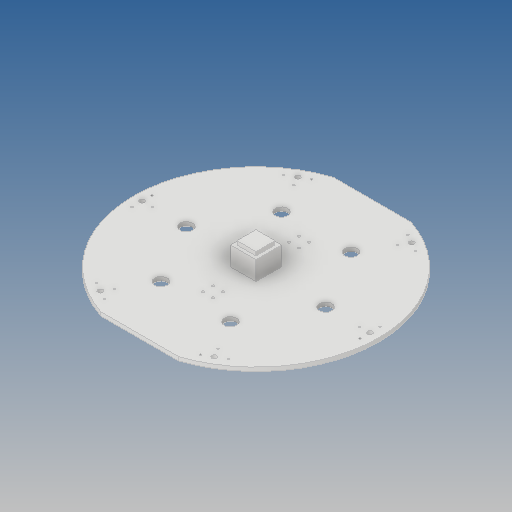
# Autodesk Inventor part: 1
Saved by Autodesk Inventor 2020 (Build 240168000, 168)
## iProperties
Created: 2019-09-06
Part Number: 1
Material: Пластик АБС
Document SubType Name: Modeling
Designer: Iliga
Density: 1.06 g/cm^3
Appearance: Гладкий — белый
Mass: 236.83 g
Surface Area: 2382.33 cm^2
Volume: 236.83 cm^3
Author: Iliga
Autodesk Inventor part; units mm, degrees
ref_plane "РабПлоскость1" through (0, -35, 0) normal (0, 1, 0) x (-1, 0, 0)
ref_plane "РабПлоскость7" through (100, -35, 0) normal (0, -1, 0) x (1, 0, 0)
sketch "Эскиз121" plane through (0, 0, 0) normal (0, 0, 1) x (1, 0, 0)
  line L0 (-100, 0) -> (0, 0)
  line L1 (0, 147.6791) -> (0, -62.3209)
  line L2 (0, 3) -> (-96.9536, 3)
  line L3 (-78.4857, 57) -> (0, 57)
  line L4 (0, 0) -> (0, 3)
  line L5 (0, 57) -> (0, 63)
  line L6 (0, 60) -> (-80, 60)
  arc A0 (-80, 60) -> (-100, 0) centre (0, 0) ccw
  arc A1 (-78.4857, 57) -> (-96.9536, 3) centre (0, 0) ccw
  dimension "d674" = 3
  dimension "d680" = 3
  dimension "d681" = 60
  dimension "d683" = 100
  dimension "d684" = 97
  constraints: 14 end point, 4 point on circle, 3 horizontal, 2 centre point, 2 coincident, 2 perpendicular, 2 point on line, 1 collinear, 1 midpoint, 1 parallel, 1 vertical
  measures "d674" distance between parallel lines of L0 L2
  measures "d680" distance between parallel lines of L3 L6
  measures "d681" distance between parallel lines of L0 L6
  measures "d683" radius of A0
  measures "d684" radius of A1
revolve "Вращение3" add sketch "Эскиз121" angle 180 mid plane about axis through (0, 147.6791, 0) along (0, -1, 0) contours A0 L6 L1 L3 A1 L2 L0
sketch "Эскиз124" plane through (0, 60, 0) normal (0, 1, 0) x (1, 0, 0)
  line L0 (-16, 50) -> (16, 50) construction
  line L1 (-16, 42) -> (16, 42)
  line L2 (16, 58) -> (-16, 58)
  arc A0 (-16, 58) -> (-16, 42) centre (-16, 50) ccw
  arc A1 (16, 42) -> (16, 58) centre (16, 50) ccw
  line L3 (0, -80) -> (0, 80) projected
  point P0 (0, 0)
  point P1 (0, 50)
  point P2 (0, 0)
  dimension "d685" = 16
  dimension "d686" = 32
  dimension "d687" = 50
  constraints: 8 end point, 4 point on circle, 4 tangent, 2 centre point, 2 midpoint, 1 horizontal, 1 parallel, 1 vertical alignment
  measures "d685" distance between parallel lines of L1 L2
  measures "d686" distance of L0.start L0.end
  measures "d687" distance of point (0, 0) point (0, 50)
extrude "Выдавливание106" cut sketch "Эскиз124" against normal blind 2.5
sketch "Эскиз125" plane through (0, 60, 0) normal (0, 1, 0) x (1, 0, 0)
  line L0 (-16, -50) -> (16, -50) construction
  line L1 (-16, -58) -> (16, -58)
  line L2 (16, -42) -> (-16, -42)
  arc A0 (-16, -42) -> (-16, -58) centre (-16, -50) ccw
  arc A1 (16, -58) -> (16, -42) centre (16, -50) ccw
  line L3 (0, -80) -> (0, 42) projected
  line L4 (0, -58) -> (0, -42)
  point P0 (0, 0)
  point P1 (0, -50)
  dimension "d690" = 16
  dimension "d691" = 32
  dimension "d692" = 50
  constraints: 10 end point, 4 point on circle, 4 tangent, 3 midpoint, 2 centre point, 2 point on line, 1 horizontal, 1 parallel, 1 vertical alignment
  measures "d690" distance between parallel lines of L1 L2
  measures "d691" distance of L0.start L0.end
  measures "d692" distance of point (0, 0) point (0, -50)
extrude "Выдавливание107" add sketch "Эскиз125" against normal blind 2.5 contours L3 L2 A1 L1
sketch "Эскиз126" plane through (0, 60, 0) normal (0, 1, 0) x (1, 0, 0)
  arc A0 (16, -58) -> (16, -42) centre (16, -50) ccw projected
  arc A1 (-16, 58) -> (-16, 42) centre (-16, 50) ccw projected
  point P0 (0, 0)
  constraints: 2 coincident
hole "Отверстие2" at (16, 60, 50) at (-16, 60, -50) direction (0, -1, 0) diameter 6.917 depth 21.1 thread size "M8x1" class "6H" standard "ISO Metric profile"
sketch "Эскиз127" plane through (0, 3, 0) normal (0, 1, 0) x (1, 0, 0)
  circle A0 centre (0, 0) radius 97 construction
  line L0 (-30.8794, 91.9536) -> (0, 91.9536)
  line L1 (0, 96.9536) -> (0, 78.4857) projected
  line L2 (-30.8794, -91.9536) -> (0, -91.9536)
  arc A1 (0, 96.9536) -> (-30.8794, 91.9536) centre (-0.863, 4.4296) ccw
  line L3 (0, -96.9536) -> (0, -78.4857) projected
  arc A2 (-30.8794, -91.9536) -> (0, -96.9536) centre (-0.8523, -4.3638) ccw
  point P0 (0, 0)
  dimension "d702" = 5
  constraints: 6 point on circle, 4 end point, 2 centre point, 2 horizontal, 1 parallel, 1 point on line, 1 vertical alignment
  measures "d702" distance from line of L1.start L0
extrude "Выдавливание108" add sketch "Эскиз127" along normal blind 20
sketch "Эскиз128" plane through (-30.7333, 3, 91.9536) normal (0, 1, 0) x (1, 0, 0)
  arc A0 (30.7333, 191.9536) -> (30.7333, -8.0464) centre (30.7333, 91.9536) ccw projected
  line L0 (30.7333, 91.9536) -> (-35.2452, -22.3245) construction
  line L1 (-32.7821, 24.7012) -> (2.9493, 4.0717) construction
  line L2 (-21.1949, 18.0113) -> (-19.9628, 20.1455) construction
  line L3 (-18.2667, 7.0831) -> (-18.9318, 7.4671) construction
  point P0 (30.7333, 91.9536)
  point P1 (-59.2667, 91.9536)
  point P2 (-14.2667, 14.0113)
  point P3 (-14.2667, 169.8959)
  point P4 (-7.3385, 10.0113)
  point P5 (-10.2667, 20.9395)
  point P6 (-59.2667, 99.9536)
  point P7 (-67.2667, 91.9536)
  point P8 (-59.2667, 83.9536)
  point P9 (-51.2667, 91.9536)
  point P10 (-7.3385, 173.8959)
  point P11 (-18.2667, 176.8241)
  point P12 (-21.1949, 165.8959)
  point P13 (-10.2667, 162.9677)
  dimension "d705" = 90
  dimension "d708" = 60
  dimension "d712" = 60
  dimension "d798" = 16
  dimension "d799" = 8
  dimension "d800" = 16
  dimension "d801" = 8
  dimension "d804" = 120
  constraints: 8 end point, 6 point on line, 3 perpendicular, 1 horizontal alignment, 13 other
  measures "d705" distance of point (30.733, 91.954) point (-59.267, 91.954)
  measures "d798" distance from line of point (-7.338, 10.011) L2
  measures "d799" distance from line of point (-14.267, 14.011) L2
  measures "d800" distance from line of point (-10.267, 20.94) L3
  measures "d801" distance from line of point (-14.267, 14.011) L3
hole "Отверстие3" at (-90, 3, 0) at (-45, 3, 77.9423) at (-45, 3, -77.9423) direction (0, -1, 0) diameter 4 depth 21.1
sketch "Эскиз129" plane through (-30.7333, 3, 91.9536) normal (0, 1, 0) x (1, 0, 0)
  point P0 (30.7333, 91.9536)
  point P1 (30.7333, 91.9536)
  point P2 (26.7333, 53.9536)
  point P3 (26.7333, 61.9536)
  point P4 (26.7333, 121.9536)
  point P5 (26.7333, 129.9536)
  dimension "d721" = 30
  dimension "d722" = 30
  dimension "d723" = 8
  dimension "d725" = 8
  dimension "d726" = 4
  constraints: 5 vertical alignment, 1 coincident
  measures "d721" vertical distance of point (30.733, 91.954) point (26.733, 61.954)
  measures "d722" vertical distance of point (30.733, 91.954) point (26.733, 121.954)
  measures "d723" distance of point (26.733, 61.954) point (26.733, 53.954)
  measures "d725" distance of point (26.733, 121.954) point (26.733, 129.954)
  measures "d726" horizontal distance of point (30.733, 91.954) point (26.733, 61.954)
hole "Отверстие4" at (-4, 3, -38) at (-4, 3, -30) at (-4, 3, 30) at (-4, 3, 38) direction (0, -1, 0) diameter 2 depth 21.1
sketch "Эскиз130" plane through (-30.7333, 3, 91.9536) normal (0, 1, 0) x (1, 0, 0)
  circle A0 centre (-59.2667, 91.9536) radius 2 projected
  arc A1 (30.7333, 191.9536) -> (30.7333, -8.0464) centre (30.7333, 91.9536) ccw projected
  point P0 (30.7333, 91.9536)
  point P1 (-24.2667, 91.9536)
  point P2 (3.2333, 44.3222)
  point P3 (3.2333, 139.585)
  dimension "d746" = 35
  dimension "d749" = 60
  dimension "d753" = 60
  constraints: 1 horizontal alignment, 4 other
  measures "d746" distance of point (-24.267, 91.954) A0.centre
hole "Отверстие5" at (-27.5, 3, -47.6314) at (-27.5, 3, 47.6314) at (-55, 3, 0) direction (0, -1, 0) diameter 10 depth 21.1
hole "Отверстие6" at (-51.9282, 3, 73.9423) at (-38.0718, 3, 81.9423) at (-49, 3, 84.8705) at (-41, 3, 71.0141) at (-90, 3, -8) at (-98, 3, 0) at (-90, 3, 8) at (-82, 3, 0) at (-38.0718, 3, -81.9423) at (-49, 3, -84.8705) at (-51.9282, 3, -73.9423) at (-41, 3, -71.0141) direction (0, -1, 0) diameter 1.567 depth 6.3 tip angle 118 thread size "M2x0.4" class "6H" standard "ANSI Metric M Profile"
sketch "Эскиз131" plane through (0, 60, 0) normal (0, 1, 0) x (1, 0, 0)
  circle A0 centre (0, 0) radius 5
  dimension "d755" = 10
  constraints: 1 centre point, 1 coincident
  measures "d755" diameter of A0
extrude "Выдавливание109" cut sketch "Эскиз131" against normal blind 25
sketch "Эскиз132" plane through (0, 0, 0) normal (0, 0, 1) x (1, 0, 0)
  line L0 (-80, 60) -> (0, 60) projected
  circle A0 centre (-80, 60) radius 10
  circle A1 centre (-80, 60) radius 8
  arc A2 (-20.6043, 23) -> (-30.7333, 3) centre (0, 0) ccw projected
  line L1 (-30.7333, 3) -> (-30.7333, 3) projected
  arc A3 (-20.6043, 23) -> (-30.7333, 3) centre (0, 0) ccw projected
  line L2 (-20.6043, 23) -> (0, 23) projected
  line L3 (0, 57) -> (0, 23) projected
  line L4 (0, 57) -> (0, 57) projected
  line L5 (0, 57) -> (0, 23) projected
  line L6 (0, 23) -> (-20.6043, 23) projected
  arc A4 (-78.4857, 57) -> (-96.9536, 3) centre (0, 0) ccw projected
  line L7 (0, 0) -> (0, 60) projected
  line L8 (0, 60) -> (0, 60) projected
  line L9 (0, 0) -> (0, 60) projected
  line L10 (0, 0) -> (0, 0) projected
  line L11 (-78.4857, 57) -> (0, 57) projected
  line L12 (-72.5838, 57) -> (-70.4606, 57)
  line L13 (-82, 52.254) -> (-83.3842, 50.59)
  point P0 (0, 0)
  dimension "d758" = 20
  dimension "d759" = 16
  dimension "d762" = 1.664
  dimension "d763" = 82
  constraints: 4 end point, 4 point on circle, 2 centre point, 2 point on line, 1 coincident
  measures "d758" diameter of A0
  measures "d759" diameter of A1
  measures "d762" vertical distance of L13.start L13.end
  measures "d763" horizontal distance of A4.centre L13.start
extrude "Выдавливание110" cut sketch "Эскиз132" along normal mid plane 150 contours A1 L11 A4 | A1 A4 L11
extrude "Выдавливание111" add sketch "Эскиз132" along normal mid plane 40 contours A1 A4 A0 L13 | L11 A0 A4 A1
sketch "Эскиз133" plane through (0, 0, 20) normal (0, 0, 1) x (1, 0, 0)
  arc A0 (-80.6647, 50.0221) -> (-70.4606, 57) centre (-80, 60) ccw projected
  arc A1 (-80.6647, 50.0221) -> (-70.4606, 57) centre (-80, 60) ccw
  line L0 (-71.9925, 60) -> (-70.4606, 57)
  arc A2 (-79.3887, 52.0234) -> (-80.6647, 50.0221) centre (0, 0) ccw projected
  arc A3 (-79.3887, 52.0234) -> (-72.5838, 57) centre (-80, 60) ccw projected
  line L1 (-72, 60) -> (0, 60) projected
  arc A4 (-79.3887, 52.0234) -> (-72, 60) centre (-80, 60) ccw
  arc A5 (-79.3887, 52.0234) -> (-80.6647, 50.0221) centre (-73.3358, 46.7568) ccw
  point P0 (0, 0)
  dimension "d768" = 3
  dimension "d773" = 10
  dimension "d774" = 8.0234
  constraints: 6 point on circle, 3 centre point, 2 end point, 1 coincident
  measures "d768" vertical distance of L0.start L0.end
  measures "d773" radius of A0
  measures "d774" radius of A5
extrude "Выдавливание113" add sketch "Эскиз133" along normal blind 11 and the other way blind 51 contours A2 A3 A4 L1 L0 A0
sketch "Эскиз134" plane through (-16, 60, -42) normal (0, 1, 0) x (1, 0, 0)
  circle A0 centre (-53, -42) radius 1.5
  line L0 (-56, -7.1288) -> (-56, -76.8712) projected
  point P0 (16, -42)
  dimension "d779" = 3
  dimension "d780" = 3
  constraints: 1 centre point, 1 horizontal alignment
  measures "d779" diameter of A0
  measures "d780" distance from line of L0 A0.centre
extrude "Выдавливание114" cut sketch "Эскиз134" against normal up to surface (3 mm away)
ref_plane "РабПлоскость27" through (-90, 0, 0) normal (1, 0, 0) x (0, 1, 0)
sketch "Эскиз135" plane through (-90, 0, 0) normal (1, 0, 0) x (0, 1, 0)
  circle A0 centre (50, 0) radius 1.5
  line L0 (60, -34.8712) -> (60, 34.8712) projected
  point P0 (0, 0)
  dimension "d784" = 3
  dimension "d785" = 10
  constraints: 1 centre point, 1 horizontal alignment, 1 vertical alignment
  measures "d784" diameter of A0
  measures "d785" distance from line of A0.centre L0
extrude "Выдавливание115" cut sketch "Эскиз135" along normal up to surface
sketch "Эскиз136" plane through (-30.7333, 3, 91.9536) normal (0, 1, 0) x (1, 0, 0)
  arc A0 (30.7333, 191.9536) -> (30.7333, -8.0464) centre (30.7333, 91.9536) ccw projected
  circle A1 centre (3.2333, 44.3222) radius 5 projected
  circle A2 centre (3.2333, 139.585) radius 5 projected
  circle A3 centre (-24.2667, 91.9536) radius 5 projected
  circle A4 centre (26.7333, 61.9536) radius 1 projected
  circle A5 centre (26.7333, 129.9536) radius 1 projected
  circle A6 centre (26.7333, 121.9536) radius 1 projected
  circle A7 centre (26.7333, 53.9536) radius 1 projected
  circle A8 centre (-14.2667, 14.0113) radius 2 projected
  circle A9 centre (-59.2667, 91.9536) radius 2 projected
  circle A10 centre (-14.2667, 169.8959) radius 2 projected
  line L0 (0, 0) -> (30.7333, 0) projected
  line L1 (30.7333, 0) -> (30.7333, 183.9072) projected
  line L2 (30.7333, 183.9072) -> (0, 183.9072) projected
  arc A11 (0, 183.9072) -> (0, 0) centre (30.7333, 91.9536) ccw projected
  point P0 (30.7333, 91.9536)
extrude "Выдавливание116" cut sketch "Эскиз136" against normal through all keep common part
mirror "Зеркальное отражение7" about plane through (0, 27.7792, 53.8643) normal (1, 0, 0)
sketch "Эскиз137" plane through (0, 3, 0) normal (0, 1, 0) x (1, 0, 0)
  line L0 (-10, -10) -> (10, -10)
  line L1 (10, -10) -> (10, 10)
  line L2 (10, 10) -> (-10, 10)
  line L3 (-10, 10) -> (-10, -10)
  line L4 (-10, -10) -> (10, 10) construction
  line L5 (10, -10) -> (-10, 10) construction
  point P0 (0, 0)
  dimension "d790" = 20
  dimension "d791" = 20
  constraints: 12 end point, 2 collinear, 2 midpoint, 1 perpendicular, 1 vertical
  measures "d790" distance of L2.end L1.end
  measures "d791" distance of L1.end L0.end
extrude "Выдавливание117" add sketch "Эскиз137" along normal blind 15
sketch "Эскиз138" plane through (0, 18, 0) normal (0, 1, 0) x (1, 0, 0)
  line L0 (-7.5, 7.5) -> (7.5, 7.5)
  line L1 (7.5, 7.5) -> (7.5, -7.5)
  line L2 (7.5, -7.5) -> (-7.5, -7.5)
  line L3 (-7.5, -7.5) -> (-7.5, 7.5)
  line L4 (-7.5, 7.5) -> (7.5, -7.5) construction
  line L5 (7.5, 7.5) -> (-7.5, -7.5) construction
  point P0 (0, 0)
  dimension "d794" = 15
  dimension "d795" = 15
  dimension "d12" = 100
  dimension "d14" = 17
  dimension "d26" = 5
  constraints: 12 end point, 2 midpoint, 2 parallel, 1 horizontal, 1 perpendicular
  measures "d794" distance of L1.end L2.end
  measures "d795" distance of L0.end L1.end
extrude "Выдавливание118" add sketch "Эскиз138" along normal blind 3
sketch "Эскиз6" plane through (0, -35, -85) normal (0, -1, 0) x (1, 0, 0)
  arc A0 (29.3991, 164.4544) -> (0, 170) centre (-5, 62.7941) ccw projected
  line L0 (0, 170) -> (0, 0) projected
  arc A1 (0, 0) -> (29.3991, 5.5456) centre (-5, 107.2059) ccw projected
  arc A2 (29.3991, 5.5456) -> (100, 85) centre (-5, 107.2059) ccw projected
  arc A3 (100, 85) -> (29.3991, 164.4544) centre (-5, 62.7941) ccw projected
  point P0 (0, 85)
  constraints: 4 end point, 1 horizontal, 1 point on circle, 1 vertical
sketch "Эскиз22" plane through (2, -165, 82.8837) normal (1, 0, 0) x (0, 0, -1)
  line L0 (167.8837, 130) -> (82.8837, 130) construction
  line L1 (165.8837, 130) -> (165.8837, 0)
  line L2 (-2.1163, 0) -> (167.8837, 0) construction
  line L3 (167.8837, 130) -> (167.8837, 0) construction
  line L4 (145.8837, 130) -> (145.8837, 0)
  line L5 (145.8837, 130) -> (165.8837, 130)
  line L6 (145.8837, 0) -> (165.8837, 0)
  point P0 (82.8837, 165)
  dimension "d115" = 2
  dimension "d116" = 20
  dimension "d121" = 143.8029
  dimension "d126" = 5
  dimension "d127" = 5
  dimension "d128" = 2
  dimension "d129" = 2
  dimension "d130" = 5
  dimension "d133" = 3
  dimension "d134" = 2
  dimension "d135" = 6
  constraints: 20 end point, 5 perpendicular, 4 point on circle, 3 horizontal, 2 point on line, 2 vertical
  measures "d126" distance between parallel lines of L1 L3
  measures "d127" distance between parallel lines of L0 L4
  measures "d128" distance between parallel lines of L5 L0
  measures "d129" distance of L2.end L6.end
sketch "Эскиз25" plane through (2, -165, 82.8837) normal (1, 0, 0) x (0, 0, -1)
  arc A0 (82.8837, 246.0941) -> (-2.1163, 165) centre (82.8837, 161) ccw projected
  arc A1 (82.8837, 244.0941) -> (-1.8354, 166.9802) centre (82.8837, 159) ccw
  line L0 (82.8837, 244.0941) -> (82.8837, 239.0941)
  line L1 (82.8837, 239.0941) -> (54.1445, 239.0941)
  point P0 (82.8837, 165)
  dimension "d138" = 2
  dimension "d139" = 2
  dimension "d140" = 2
  dimension "d141" = 5
  dimension "d257" = 4
  dimension "d258" = 2
  dimension "d259" = 2
  dimension "d260" = 2
  dimension "d261" = 2
  dimension "d262" = 16
  dimension "d263" = 16
  dimension "d264" = 16
  dimension "d265" = 16
  dimension "d266" = 4
  dimension "d267" = 4
  dimension "d268" = 4
  dimension "d269" = 2
  dimension "d270" = 2
  dimension "d271" = 2
  dimension "d272" = 2
  dimension "d273" = 2
  dimension "d274" = 2
  dimension "d275" = 2
  dimension "d276" = 2
  dimension "d277" = 2
  dimension "d278" = 2
  dimension "d279" = 2
  dimension "d280" = 2
  dimension "d448" = 15
  dimension "d449" = 15
  dimension "d450" = 50
  dimension "d451" = 50
  dimension "d452" = 50
  dimension "d453" = 50
  dimension "d454" = 95
  dimension "d455" = 95
  dimension "d456" = 16
  dimension "d457" = 4
  dimension "d458" = 2
  dimension "d459" = 2
  dimension "d460" = 2
  dimension "d461" = 2
  dimension "d462" = 16
  dimension "d463" = 4
  dimension "d464" = 2
  dimension "d465" = 2
  dimension "d466" = 2
  dimension "d467" = 2
  dimension "d468" = 95
  dimension "d469" = 50
  dimension "d470" = 50
  dimension "d471" = 95
  constraints: 36 centre point, 24 point on circle, 12 coincident, 12 horizontal alignment, 12 vertical alignment, 2 end point, 1 midpoint, 1 vertical
  measures "d262" diameter of A0
  measures "d263" diameter of A1
  measures "d448" distance from line of L0 point (-95, -35)
  measures "d449" distance from line of L0 point (5, -35)
  measures "d450" distance from line of L1 point (-95, -35)
  measures "d451" distance from line of L1 point (5, -35)
  measures "d452" distance from line of L1 point (-95, 60)
  measures "d453" distance from line of L1 point (5, 60)
  measures "d454" distance of point (-95, -35) point (-95, 60)
  measures "d455" distance of point (5, -35) point (5, 60)
  measures "d468" distance of point (-95, 60) point (-95, 155)
  measures "d469" distance from line of L1 point (-95, 155)
  measures "d470" distance from line of L1 point (5, 155)
  measures "d471" distance of point (5, 60) point (5, 155)
sketch "Эскиз61" plane through (0, -165, -85) normal (0, -1, 0) x (1, 0, 0)
  line L0 (63.3161, 9.7707) -> (45.9008, 9.7707)
  line L1 (45.9008, 9.7707) -> (45.9008, 31.4712)
  line L2 (45.9008, 31.4712) -> (63.3161, 31.4712)
  line L3 (63.3161, 31.4712) -> (63.3161, 9.7707)
  arc A0 (2, 2.1163) -> (45.9008, 15) centre (-5, 107.2059) ccw projected
  point P0 (0, 85)
  dimension "d431" = 10
  dimension "d432" = 10
  dimension "d503" = 47
  dimension "d504" = 15
  dimension "d505" = 15
  dimension "d508" = 30
  dimension "d515" = 95
  constraints: 8 centre point, 2 vertical, 1 horizontal alignment, 12 other
sketch "Эскиз87" plane through (0, -35, 85) normal (-1, 0, 0) x (0, 0, 1)
  circle A0 centre (-89, -71.5) radius 1
  line L0 (0, -130) -> (-170, -130) projected
  circle A1 centre (-81, -71.5) radius 1
  line L1 (0, -130) -> (-170, -130) projected
  line L2 (-81.4837, -130) -> (-88.5163, -130) projected
  line L3 (-85, -130) -> (-85, 95) construction
  line L4 (-81, -71.5) -> (-89, -71.5) construction
  circle A2 centre (-89, -63.5) radius 1
  circle A3 centre (-81, -63.5) radius 1
  circle A4 centre (-81, 23.5) radius 1
  circle A5 centre (-81, 31.5) radius 1
  circle A6 centre (-89, 23.5) radius 1
  circle A7 centre (-89, 31.5) radius 1
  circle A8 centre (-89, -71.5) radius 1 projected
  circle A9 centre (-89, 23.5) radius 1 projected
  point P0 (-88.3838, -130)
  point P1 (-119.3064, -130)
  point P2 (-50.6936, -130)
  point P3 (-81.6162, -130)
  point P4 (-85, -71.5)
  dimension "d479" = 2
  dimension "d481" = 2
  dimension "d483" = 8
  dimension "d486" = 8
  dimension "d491" = 2
  dimension "d495" = 8
  dimension "d498" = 8
  dimension "d638" = 87
  constraints: 8 centre point, 4 end point, 3 midpoint, 3 vertical, 2 vertical alignment, 1 coincident, 1 horizontal, 10 other
  measures "d479" diameter of A0
  measures "d481" diameter of A1
  measures "d483" distance of L4.start L4.end
  measures "d486" distance of L4.end A2.centre
  measures "d491" diameter of A4
  measures "d495" distance of A4.centre A5.centre
  measures "d498" distance of A4.centre A6.centre
  measures "d638" distance of A3.centre A4.centre
sketch "Эскиз109" plane through (100, -36, 0) normal (0, 1, 0) x (1, 0, 0)
  line L0 (-54.0992, 63) -> (-98, 63) projected
  line L1 (-98, 0) -> (-98, 82.8837) projected
  line L2 (-70, 63) -> (-68, 63)
  line L3 (-68, 63) -> (-68, 60)
  line L4 (-68, 60) -> (-70, 60)
  line L5 (-70, 60) -> (-70, 63)
  line L6 (-65.5, 63) -> (-63.5, 63)
  line L7 (-63.5, 63) -> (-63.5, 60)
  line L8 (-63.5, 60) -> (-65.5, 60)
  line L9 (-65.5, 60) -> (-65.5, 63)
  point P0 (-100, 0)
  dimension "d588" = 30
  dimension "d589" = 2
  dimension "d590" = 2
  dimension "d591" = 2.5
  dimension "d592" = 3
  constraints: 16 end point, 4 parallel, 2 horizontal, 2 perpendicular, 2 point on line, 1 horizontal alignment
  measures "d588" distance of L0.end L2.end
  measures "d589" distance between parallel lines of L3 L5
  measures "d590" distance between parallel lines of L7 L9
  measures "d591" distance between parallel lines of L3 L9
  measures "d592" distance of L2.start L4.end
sketch "Эскиз110" plane through (0, -165, -85) normal (0, -1, 0) x (1, 0, 0)
  arc A0 (97.9549, 85) -> (2, 167.8837) centre (-5, 62.7941) ccw projected
  line L0 (97.9395, 85) -> (14.2936, 85) projected
  line L1 (30, 22) -> (30, 25) projected
  line L2 (32, 25) -> (32, 22) projected
  line L3 (34.5, 22) -> (34.5, 25) projected
  line L4 (36.5, 25) -> (36.5, 22) projected
  line L5 (30, 85) -> (30, 162.131)
  line L6 (32, 85) -> (32, 161.4035)
  line L7 (34.5, 85) -> (34.5, 160.429)
  line L8 (36.5, 85) -> (36.5, 159.5958)
  point P0 (0, 85)
  point P1 (2, 167.8837)
  point P2 (18.2297, 165.5228)
  point P3 (50.539, 152.2828)
  point P4 (97.9549, 85)
  point P5 (30, 23.5)
  point P6 (32, 23.5)
  point P7 (34.5, 23.5)
  point P8 (36.5, 23.5)
  constraints: 8 end point, 4 midpoint, 4 point on line, 4 vertical alignment, 3 vertical, 1 parallel, 7 other
sketch "Эскиз111" plane through (36.5, -165, 74.5958) normal (1, 0, 0) x (0, 0, -1)
  line L0 (74.5958, 0) -> (74.5958, 228.8154) projected
  line L1 (-0.8332, 0) -> (74.5958, 0) projected
  line L2 (-0.8332, 144.6272) -> (-0.8332, 0) projected
  line L3 (2.1668, 0) -> (2.1668, 144.6272)
  arc A0 (74.5958, 225.8154) -> (2.1668, 144.6272) centre (84.7947, 143.8154) ccw
  line L4 (2.1668, 0) -> (74.5958, 0)
  line L5 (74.5958, 0) -> (74.5958, 225.8154)
  point P0 (74.5958, 165)
  dimension "d597" = 3
  dimension "d598" = 3
  dimension "d599" = 85
  constraints: 6 end point, 2 point on circle, 1 centre point, 1 collinear, 1 horizontal alignment, 1 perpendicular, 1 point on line, 1 vertical, 1 other
  measures "d597" distance between parallel lines of L2 L3
  measures "d598" distance of L0.end L5.end
  measures "d599" vertical distance of L0.end A0.centre
sketch "Эскиз114" plane through (2, -165, 82.8837) normal (1, 0, 0) x (0, 0, -1)
  circle A0 centre (120.1897, 5) radius 1
  line L0 (-2.1163, 0) -> (167.8837, 0) construction
  line L1 (82.8837, 0) -> (82.8837, 60.2174) construction
  circle A1 centre (45.5777, 5) radius 1
  point P0 (82.8837, 165)
  dimension "d609" = 2
  dimension "d610" = 37.306
  dimension "d611" = 5
  constraints: 2 centre point, 2 end point, 1 midpoint, 1 symmetric about line, 1 vertical, 1 other
  measures "d609" diameter of A0
  measures "d610" distance from line of L1 A0.centre
  measures "d611" distance from line of L0 A0.centre
sketch "Эскиз117" plane through (2, -165, 82.8837) normal (1, 0, 0) x (0, 0, -1)
  circle A0 centre (104.8837, 10) radius 1
  line L0 (145.8837, 0) -> (0, 0) construction
  line L1 (82.8837, 130) -> (82.8837, 0) construction
  circle A1 centre (60.8837, 10) radius 1
  point P0 (82.8837, 165)
  dimension "d624" = 2
  dimension "d625" = 10
  dimension "d626" = 22
  dimension "d629" = 2
  dimension "d631" = 22
  dimension "d632" = 10
  constraints: 2 centre point
  measures "d624" diameter of A0
  measures "d625" distance from line of L0 A0.centre
  measures "d626" distance from line of L1 A0.centre
  measures "d629" diameter of A1
  measures "d631" distance from line of L1 A1.centre
  measures "d632" distance from line of L0 A1.centre
sketch "Эскиз118" plane through (100, -165, 0) normal (1, 0, 0) x (0, 0, -1)
  line L0 (-85, 0) -> (0, 0) projected
  line L1 (0, 130) -> (0, 0) projected
  circle A0 centre (-9.5, 10) radius 1
  point P0 (0, 165)
  dimension "d633" = 2
  dimension "d634" = 9.5
  dimension "d635" = 10
  constraints: 1 centre point
  measures "d633" diameter of A0
  measures "d634" distance from line of L1 A0.centre
  measures "d635" distance from line of L0 A0.centre
sketch "Эскиз119" plane through (82, -165, -85) normal (-1, 0, 0) x (0, 0, 1)
  line L0 (170, 0) -> (0, 0) projected
  line L1 (0, 0) -> (175, 0)
  line L2 (175, 0) -> (175, 251)
  line L3 (175, 251) -> (0, 251)
  line L4 (0, 251) -> (0, 0)
  point P0 (85, 165)
  dimension "d640" = 251
  dimension "d641" = 175
  constraints: 8 end point, 2 parallel, 1 horizontal, 1 perpendicular
  measures "d640" distance of L1.end L2.end
  measures "d641" distance of L2.end L3.end
sketch "Эскиз120" plane through (0, -165, -85) normal (-1, 0, 0) x (0, 0, 1)
  line L0 (170, 0) -> (0, 0) projected
  arc A0 (0, 0) -> (170, 0) centre (85, 52.6783) ccw
  point P0 (85, 165)
  dimension "d649" = 100
  dimension "d10" = 170
  dimension "d15" = 4
  dimension "d16" = 35
  dimension "d97" = 2
  constraints: 10 end point, 3 point on circle, 2 horizontal, 2 vertical alignment, 1 centre point, 1 horizontal alignment, 1 perpendicular, 1 vertical
  measures "d10" distance of L0.start L0.end
  measures "d15" distance of point (0, 0) A0.centre
